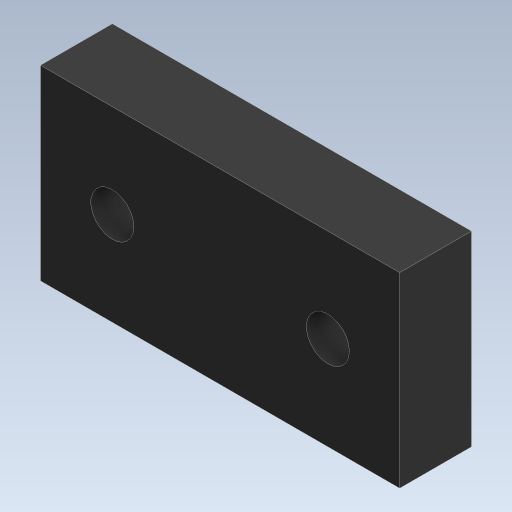
# Autodesk Inventor part: alza
Saved by Autodesk Inventor 2023 (Build 270158000, 158)
## iProperties
Created: 2023-03-26
Part Number: alza
Material: Rubber, Silicone
Document SubType Name: Modeling
Designer: santi
Density: 1.25 g/cm^3
Appearance: Rubber - Black
Author: santi
Autodesk Inventor part; units mm, degrees
ref_plane "YZ Plane" through (0, 0, 0) normal (1, 0, 0) x (0, 1, 0)
ref_plane "XZ Plane" through (0, 0, 0) normal (0, 1, 0) x (-1, 0, 0)
ref_plane "XY Plane" through (0, 0, 0) normal (0, 0, 1) x (1, 0, 0)
sketch "Sketch1" plane through (0, 0, 0) normal (0, 0, 1) x (1, 0, 0)
  line L0 (0, 0) -> (25, 0)
  line L1 (25, 0) -> (25, 13)
  line L2 (25, 13) -> (0, 13)
  line L3 (0, 13) -> (0, 0)
  circle A0 centre (5, 6.5) radius 1.5
  circle A1 centre (20, 6.5) radius 1.5
  point P0 (25, 6.5)
  dimension "d0" = 25
  dimension "d1" = 3
  dimension "d2" = 3
  dimension "d3" = 15
  dimension "d4" = 5
  dimension "d5" = 13
  constraints: 8 end point, 2 centre point, 2 horizontal alignment, 2 parallel, 1 horizontal, 1 midpoint, 1 perpendicular
  measures "d0" distance of L1.end L2.end
  measures "d1" diameter of A0
  measures "d2" diameter of A1
  measures "d3" distance of A1.centre A0.centre
  measures "d4" distance from line of L1 A1.centre
  measures "d5" distance of L0.end L1.end
extrude "Extrusion1" add sketch "Sketch1" along normal blind 5
body "Solid1"
